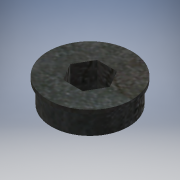
# Autodesk Inventor part: hex bearing
Saved by Autodesk Inventor 2016 (Build 200138000, 138)
## iProperties
Created: 2016-01-17
Part Number: hex bearing
Material: Steel
Document SubType Name: Modeling
Designer: gus
Density: 7.85 g/cm^3
Appearance: Plate
Mass: 38.0312 g
Surface Area: 24.9709 cm^2
Volume: 4.84474 cm^3
User Status: complete
Author: gus
Autodesk Inventor part; units mm, degrees
ref_plane "YZ Plane" through (0, 0, 0) normal (1, 0, 0) x (0, 1, 0)
ref_plane "XZ Plane" through (0, 0, 0) normal (0, 1, 0) x (-1, 0, 0)
ref_plane "XY Plane" through (0, 0, 0) normal (0, 0, 1) x (1, 0, 0)
sketch "Sketch1" plane through (0, 0, 0) normal (0, 1, 0) x (-1, 0, 0)
  circle A0 centre (0, 0) radius 14.2875
  line L0 (3.6662, 6.35) -> (7.3323, 0)
  line L1 (7.3323, 0) -> (3.6662, -6.35)
  line L2 (3.6662, -6.35) -> (-3.6662, -6.35)
  line L3 (-3.6662, -6.35) -> (-7.3323, 0)
  line L4 (-7.3323, 0) -> (-3.6662, 6.35)
  line L5 (-3.6662, 6.35) -> (3.6662, 6.35)
  dimension "d0" = 28.575
  dimension "d1" = 12.7
  constraints: 12 end point, 2 coincident, 1 centre point, 1 horizontal, 13 other
  measures "d0" diameter of A0
  measures "d1" distance between parallel lines of L2 L5
extrude "Extrusion1" add sketch "Sketch1" along normal blind 7.7724
sketch "Sketch2" plane through (0, 7.7724, 0) normal (0, 1, 0) x (1, 0, 0)
  circle A0 centre (0, 0) radius 15.5575
  line L0 (-3.6662, 6.35) -> (3.6662, 6.35) projected
  line L1 (-3.6662, 6.35) -> (3.6662, 6.35)
  line L2 (3.6662, 6.35) -> (7.3323, 0)
  line L3 (7.3323, 0) -> (3.6662, -6.35)
  line L4 (3.6662, -6.35) -> (-3.6662, -6.35)
  line L5 (-3.6662, -6.35) -> (-7.3323, 0)
  line L6 (-7.3323, 0) -> (-3.6662, 6.35)
  dimension "d4" = 31.115
  constraints: 12 end point, 2 coincident, 1 centre point, 13 other
  measures "d4" diameter of A0
extrude "Extrusion2" add sketch "Sketch2" along normal blind 1.524
body "Solid1"
